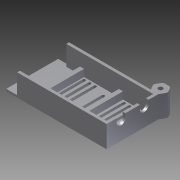
# Autodesk Inventor part: case add on sdr botom
Saved by Autodesk Inventor 2012 (Build 160160000, 160)
## iProperties
Created: 2018-03-03
Part Number: case add on sdr botom
Material: Default
Document SubType Name: Modeling
Designer: kanu
Density: 1 g/cm^3
Author: kanu
Autodesk Inventor part; units mm, degrees
ref_plane "YZ Plane" through (0, 0, 0) normal (1, 0, 0) x (0, 1, 0)
ref_plane "XZ Plane" through (0, 0, 0) normal (0, 1, 0) x (-1, 0, 0)
ref_plane "XY Plane" through (0, 0, 0) normal (0, 0, 1) x (1, 0, 0)
sketch "Sketch1" plane through (0, 0, 0) normal (0, 0, 1) x (1, 0, 0)
  line L0 (-79.2915, 39.2514) -> (-13.7915, 39.2514)
  line L1 (-13.7915, 39.2514) -> (-13.7915, 1.2514)
  line L2 (-13.7915, 1.2514) -> (-79.2915, 1.2514)
  line L3 (-79.2915, 1.2514) -> (-79.2915, 39.2514)
  point P0 (0, 0)
  constraints: 8 end point, 2 parallel, 1 horizontal, 1 perpendicular
extrude "Extrusion1" add sketch "Sketch1" along normal blind 1.5
sketch "Sketch2" plane through (0, 0, 1.5) normal (0, 0, 1) x (1, 0, 0)
  line L0 (-13.7915, 39.2514) -> (-13.7915, 1.2514) projected
  line L1 (-79.2915, 39.2514) -> (-13.7915, 39.2514) projected
  line L2 (-79.2915, 1.2514) -> (-79.2915, 39.2514) projected
  line L3 (-13.7915, 1.2514) -> (-79.2915, 1.2514) projected
  line L4 (-79.2915, 37.2514) -> (-15.7915, 37.2514)
  line L5 (-15.7915, 37.2514) -> (-15.7915, 3.2514)
  line L6 (-15.7915, 3.2514) -> (-79.2915, 3.2514)
  point P0 (0, 0)
  dimension "d2" = 2
  dimension "d3" = 2
  dimension "d4" = 2
  constraints: 6 end point, 3 perpendicular, 2 point on line
  measures "d2" distance between parallel lines of L1 L4
  measures "d3" distance between parallel lines of L5 L0
  measures "d4" distance between parallel lines of L3 L6
extrude "Extrusion2" add sketch "Sketch2" along normal blind 14.5 contours L0 L3 L2 L6 L5 L4 L1
sketch "Sketch3" plane through (-13.7915, 1.2514, 0) normal (1, 0, 0) x (0, 0, -1)
  line L0 (0, 0) -> (-16, 0) projected
  line L1 (0, 38) -> (0, 0) projected
  line L2 (0, 38) -> (-16, 38) projected
  line L3 (-16, 38) -> (-16, 0) projected
  arc A0 (-13, 24.3) -> (-13, 30.7) centre (-13, 27.5) ccw
  line L4 (-13, 30.7) -> (-16, 30.7)
  line L5 (-13, 24.3) -> (-16, 24.3)
  arc A1 (-13, 7.3) -> (-13, 13.7) centre (-13, 10.5) ccw
  line L6 (-13, 7.3) -> (-16, 7.3)
  line L7 (-13, 13.7) -> (-16, 13.7)
  point P0 (0, -1.2514)
  dimension "d7" = 13
  dimension "d8" = 10.5
  dimension "d9" = 3.2
  dimension "d10" = 13
  dimension "d11" = 10.5
  constraints: 8 end point, 4 point on circle, 4 point on line, 4 tangent, 2 centre point, 2 parallel, 2 perpendicular
  measures "d7" distance from line of L1 A0.centre
  measures "d8" distance from line of L2 A0.centre
  measures "d9" radius of A0
  measures "d10" distance from line of L1 A1.centre
  measures "d11" distance from line of L0 A1.centre
extrude "Extrusion3" cut sketch "Sketch3" against normal blind 13 contours L3 L7 A1 L6 | L4 A0 L5 L3
sketch "Sketch4" plane through (0, 0, 0) normal (0, 0, -1) x (-1, 0, 0)
  line L0 (21.3312, 42.5198) -> (19.2419, 38.901)
  arc A0 (21.3312, 42.5198) -> (21.3312, 44.5198) centre (19.5992, 43.5198) ccw
  line L1 (19.8192, 47.1386) -> (21.3312, 44.5198)
  arc A1 (19.8192, 47.1386) -> (18.0872, 48.1386) centre (18.0872, 46.1386) ccw
  line L2 (15.0633, 48.1386) -> (18.0872, 48.1386)
  arc A2 (15.0633, 48.1386) -> (13.3312, 47.1386) centre (15.0633, 46.1386) ccw
  line L3 (11.8192, 44.5198) -> (13.3312, 47.1386)
  arc A3 (11.8192, 44.5198) -> (11.8192, 42.5198) centre (13.5513, 43.5198) ccw
  line L4 (12.8585, 40.7198) -> (11.8192, 42.5198)
  circle A4 centre (16.5752, 43.5198) radius 1.65
  line L5 (12.8585, 40.7198) -> (13.7938, 39.0998)
  line L6 (13.7938, 39.0998) -> (19.3567, 39.0998)
  point P0 (0, 0)
  point P1 (16.0419, 38.7198)
  constraints: 14 end point, 8 point on circle, 5 centre point, 2 parallel, 1 point on line
extrude "Extrusion4" add sketch "Sketch4" against normal blind 16
sketch "Sketch5" plane through (-79.2915, 1.2514, 0) normal (-1, 0, 0) x (0, 0, 1)
  line L0 (1.5, 2) -> (1.5, 36) projected
  line L1 (0, 38) -> (16, 38) projected
  line L2 (0, 0) -> (0, 38) projected
  line L3 (0, 0) -> (16, 0) projected
  line L4 (1.5, 36) -> (1.5, 38)
  line L5 (1.5, 2) -> (1.5, 0)
  point P0 (0, -1.2514)
  constraints: 4 end point, 2 perpendicular, 2 point on line
extrude "Extrusion5" add sketch "Sketch5" along normal blind 8
sketch "Sketch6" plane through (0, 0, 1.5) normal (0, 0, 1) x (1, 0, 0)
  line L0 (-15.7915, 37.2514) -> (-79.2915, 37.2514) projected
  line L1 (-79.2915, 3.2514) -> (-15.7915, 3.2514) projected
  line L2 (-15.7915, 3.2514) -> (-15.7915, 37.2514) projected
  line L3 (-69.2915, 37.2514) -> (-66.2915, 37.2514)
  line L4 (-66.2915, 37.2514) -> (-66.2915, 3.2514)
  line L5 (-66.2915, 3.2514) -> (-69.2915, 3.2514)
  line L6 (-69.2915, 3.2514) -> (-69.2915, 37.2514)
  line L7 (-40.7915, 37.2514) -> (-37.7915, 37.2514)
  line L8 (-37.7915, 37.2514) -> (-37.7915, 3.2514)
  line L9 (-37.7915, 3.2514) -> (-40.7915, 3.2514)
  line L10 (-40.7915, 3.2514) -> (-40.7915, 37.2514)
  point P0 (0, 0)
  dimension "d18" = 3
  dimension "d19" = 3
  dimension "d20" = 22
  dimension "d21" = 10
  constraints: 16 end point, 4 parallel, 4 point on line, 2 horizontal, 2 perpendicular
  measures "d18" distance of L3.start L3.end
  measures "d19" distance of L7.start L7.end
  measures "d20" distance between parallel lines of L2 L8
  measures "d21" distance from line of L0.end L6
extrude "Extrusion6" add sketch "Sketch6" along normal blind 5.2 contours L8 L1 L10 L0 | L4 L1 L6 L0
sketch "Sketch7" plane through (0, 0, 0) normal (0, 0, -1) x (-1, 0, 0)
  line L0 (87.2915, 39.2514) -> (19.4442, 39.2514) projected
  line L1 (18.0872, 35.2514) -> (20.0872, 35.2514)
  line L2 (20.0872, 35.2514) -> (20.0872, 5.2514)
  line L3 (20.0872, 5.2514) -> (18.0872, 5.2514)
  line L4 (18.0872, 5.2514) -> (18.0872, 35.2514)
  circle A0 centre (19.0872, 35.2514) radius 1
  circle A1 centre (19.0872, 5.2514) radius 1
  point P0 (0, 0)
  dimension "d24" = 2
  dimension "d25" = 30
  dimension "d26" = 4
  dimension "d32" = 2
  dimension "d33" = 2
  constraints: 8 end point, 2 centre point, 2 midpoint, 2 parallel, 1 horizontal, 1 perpendicular
  measures "d24" distance between parallel lines of L4 L2
  measures "d25" vertical distance of L1.end A1.centre
  measures "d26" distance from line of L0 A0.centre
  measures "d32" diameter of A0
  measures "d33" diameter of A1
extrude "Extrusion7" cut sketch "Sketch7" against normal blind 2
pattern_linear "Rectangular Pattern1" count 5 spacing 4 along (-1, 0, 0) of "Extrusion7"
sketch "Sketch8" plane through (0, 0, 0) normal (0, 0, -1) x (-1, 0, 0)
  line L0 (13.7915, 1.2514) -> (87.2915, 1.2514) projected
  line L1 (87.2915, 1.2514) -> (87.2915, 39.2514) projected
  line L2 (42.2915, 32.2514) -> (44.2915, 32.2514)
  line L3 (44.2915, 32.2514) -> (44.2915, 8.2514)
  line L4 (44.2915, 8.2514) -> (42.2915, 8.2514)
  line L5 (42.2915, 8.2514) -> (42.2915, 32.2514)
  circle A0 centre (43.2915, 32.2514) radius 1
  circle A1 centre (43.2915, 8.2514) radius 1
  point P0 (0, 0)
  dimension "d34" = 2
  dimension "d35" = 24
  dimension "d36" = 43
  dimension "d37" = 7
  constraints: 8 end point, 2 centre point, 2 midpoint, 2 parallel, 1 horizontal, 1 perpendicular
  measures "d34" distance between parallel lines of L5 L3
  measures "d35" distance of L2.end L3.end
  measures "d36" distance between parallel lines of L1 L3
  measures "d37" distance between parallel lines of L0 L4
extrude "Extrusion8" cut sketch "Sketch8" against normal blind 2
pattern_linear "Rectangular Pattern2" count 2 spacing 4 along (-1, 0, 0) of "Extrusion8"
sketch "Sketch9" plane through (0, 0, 0) normal (0, 0, -1) x (-1, 0, 0)
  line L0 (87.2915, 39.2514) -> (19.4442, 39.2514) projected
  line L1 (55.3139, 35.2514) -> (57.3139, 35.2514)
  line L2 (57.3139, 35.2514) -> (57.3139, 5.2514)
  line L3 (57.3139, 5.2514) -> (55.3139, 5.2514)
  line L4 (55.3139, 5.2514) -> (55.3139, 35.2514)
  circle A0 centre (56.3139, 35.2514) radius 1
  circle A1 centre (56.3139, 5.2514) radius 1
  point P0 (0, 0)
  dimension "d43" = 30
  dimension "d44" = 4
  constraints: 8 end point, 2 centre point, 2 midpoint, 2 parallel, 1 horizontal, 1 perpendicular
  measures "d43" distance of L1.end L2.end
  measures "d44" distance between parallel lines of L0 L1
extrude "Extrusion9" cut sketch "Sketch9" against normal blind 2
pattern_linear "Rectangular Pattern3" count 3 spacing 4 along (-1, 0, 0) of "Extrusion9"
body "Solid1"
